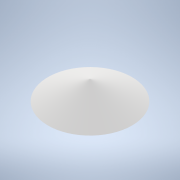
# Autodesk Inventor part: lidar lidimost
Saved by Autodesk Inventor 2022 (Build 260153000, 153)
## iProperties
Created: 2024-11-12
Part Number: lidar lidimost
Material: Типовые
Document SubType Name: Modeling
Designer: Andrey
Density: 1 g/cm^3
Appearance: По умолчанию
Author: Andrey
Autodesk Inventor part; units mm, degrees
ref_plane "YZ Plane" through (0, 0, 0) normal (1, 0, 0) x (0, 1, 0)
ref_plane "XZ Plane" through (0, 0, 0) normal (0, 1, 0) x (-1, 0, 0)
ref_plane "XY Plane" through (0, 0, 0) normal (0, 0, 1) x (1, 0, 0)
sketch "Эскиз1" plane through (0, 0, 0) normal (0, 0, 1) x (1, 0, 0)
  line L0 (0, 0) -> (249.5571, -116.3704)
  line L1 (0, 0) -> (275.3558, 0) construction
  line L2 (249.5571, -116.3704) -> (0, -116.3704)
  line L3 (0, -116.3704) -> (0, 0)
  dimension "d0" = 25
  constraints: 8 end point, 2 horizontal, 1 equal length, 1 perpendicular
  measures "d0" angle of L0 L1
revolve "Вращение1" add sketch "Эскиз1" angle 360 about axis through (0, -116.3704, 0) along (0, 1, 0)
